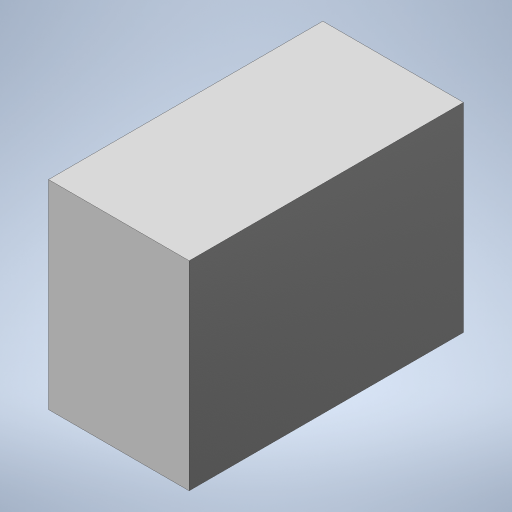
# Autodesk Inventor part: small cupboard
Saved by Autodesk Inventor 2023 (Build 270158000, 158)
## iProperties
Created: 2022-09-12
Part Number: small cupboard
Material: 常规
Document SubType Name: Modeling
Designer: byfbi
Density: 1 g/cm^3
Appearance: 默认
Author: byfbi
Autodesk Inventor part; units mm, degrees
ref_plane "YZ Plane" through (0, 0, 0) normal (1, 0, 0) x (0, 1, 0)
ref_plane "XZ Plane" through (0, 0, 0) normal (0, 1, 0) x (-1, 0, 0)
ref_plane "XY Plane" through (0, 0, 0) normal (0, 0, 1) x (1, 0, 0)
sketch "草图1" plane through (0, 0, 0) normal (1, 0, 0) x (0, 1, 0)
  line L0 (425, -600) -> (-425, -600)
  line L1 (-425, -600) -> (-425, 600)
  line L2 (-425, 600) -> (425, 600)
  line L3 (425, 600) -> (425, -600)
  line L4 (425, -600) -> (-425, 600) construction
  line L5 (-425, -600) -> (425, 600) construction
  point P0 (0, 0)
  dimension "d0" = 850
  dimension "d1" = 1200
  constraints: 12 end point, 2 midpoint, 2 parallel, 1 horizontal, 1 perpendicular
  measures "d0" distance of L1.end L2.end
  measures "d1" distance of L0.end L1.end
extrude "拉伸1" add sketch "草图1" along normal blind 600
sketch "草图2" plane through (0, -425, -600) normal (0, 0, -1) x (-1, 0, 0)
  line L0 (0, 0) -> (0, 850) projected
  line L1 (0, 850) -> (-600, 850) projected
  line L2 (-600, 0) -> (-600, 850) projected
  line L3 (0, 0) -> (-600, 0) projected
  point P0 (0, 425)
extrude "拉伸2" cut sketch "草图2" against normal blind 30
